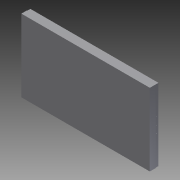
# Autodesk Inventor part: tv
Saved by Autodesk Inventor 2014 (Build 180170000, 170)
## iProperties
Created: 2014-03-21
Part Number: tv
Material: Generic
Document SubType Name: Modeling
Designer: joe_000
Density: 1 g/cm^3
Appearance: Default
largeScrewDiameter: 0.195 in
screwDistanceFromBack: 0.641 in
largeScrewDistance: 5.875 in
topLargeScrewDistanceFromTop: 11.750 in
Author: joe_000
Autodesk Inventor part; units mm, degrees
ref_plane "YZ Plane" through (0, 0, 0) normal (1, 0, 0) x (0, 1, 0)
ref_plane "XZ Plane" through (0, 0, 0) normal (0, 1, 0) x (-1, 0, 0)
ref_plane "XY Plane" through (0, 0, 0) normal (0, 0, 1) x (1, 0, 0)
sketch "Sketch1" plane through (0, 0, 0) normal (0, 0, 1) x (1, 0, 0)
  line L0 (0, 0) -> (1339.85, 0)
  line L1 (1339.85, 0) -> (1339.85, 755.65)
  line L2 (1339.85, 755.65) -> (0, 755.65)
  line L3 (0, 755.65) -> (0, 0)
  dimension "tvWidth" = 1339.85
  dimension "tvHeight" = 755.65
  dimension "tvDiagonal" = 1538.2474
  constraints: 8 end point, 2 parallel, 1 horizontal, 1 perpendicular
  measures "tvWidth" distance of L1.end L2.end
  measures "tvHeight" distance of L0.end L1.end
  measures "tvDiagonal" distance of L1.end L0.start
extrude "Extrusion1" add sketch "Sketch1" against normal blind 59.9281
sketch "Sketch2" plane through (0, 0, -59.9281) normal (0, 0, -1) x (-1, 0, 0)
  line L0 (-1339.85, 0) -> (-1339.85, 755.65) projected
  line L1 (0, 0) -> (-1339.85, 0) projected
  line L2 (0, 755.65) -> (0, 0) projected
  line L3 (-1339.85, 755.65) -> (0, 755.65) projected
  line L4 (-1337.8656, 753.6656) -> (-1.9844, 753.6656)
  line L5 (-1.9844, 753.6656) -> (-1.9844, 1.9844)
  line L6 (-1.9844, 1.9844) -> (-1337.8656, 1.9844)
  line L7 (-1337.8656, 1.9844) -> (-1337.8656, 753.6656)
  dimension "backBezelToFrontBezelSizeDifference" = 1.9844
  dimension "d7" = 1.9844
  dimension "d8" = 1.9844
  dimension "d9" = 1.9844
  constraints: 8 end point, 2 parallel, 1 horizontal, 1 perpendicular
  measures "backBezelToFrontBezelSizeDifference" distance between parallel lines of L2 L5
  measures "d7" distance between parallel lines of L3 L4
  measures "d8" distance between parallel lines of L0 L7
  measures "d9" distance between parallel lines of L1 L6
extrude "Extrusion2" add sketch "Sketch2" along normal blind 32.1469 contours L4 L5 L6 L7
sketch "Sketch3" plane through (1337.8656, 1.9844, -59.9281) normal (1, 0, 0) x (0, 0, -1)
  line L0 (32.1469, 0) -> (32.1469, 751.6812) projected
  line L1 (0, 751.6812) -> (32.1469, 751.6812) projected
  circle A0 centre (15.875, 453.2312) radius 2.4805
  circle A1 centre (15.875, 304.0062) radius 2.4805
  circle A2 centre (15.875, 378.4203) radius 1.6867
  point P0 (-59.9281, -1.9844)
  dimension "largeScrewDistance" = 149.225
  dimension "largeScrewToSmallScrewDistance" = 74.8109
  dimension "screwDistanceFromBack" = 16.2719
  dimension "topLargeScrewDistanceFromTop" = 298.45
  dimension "largeScrewDiameter" = 4.9609
  dimension "smallScrewDiameter" = 3.3734
  constraints: 3 centre point, 2 vertical alignment, 1 equal radius
  measures "largeScrewDistance" distance of A0.centre A1.centre
  measures "largeScrewToSmallScrewDistance" distance of A2.centre A0.centre
  measures "screwDistanceFromBack" distance from line of L0 A0.centre
  measures "topLargeScrewDistanceFromTop" distance from line of L1 A0.centre
  measures "largeScrewDiameter" diameter of A0
  measures "smallScrewDiameter" diameter of A2
extrude "Extrusion3" cut sketch "Sketch3" against normal blind 18.2563
equation "\"d7\" = backBezelToFrontBezelSizeDifference"
equation "\"d8\" = backBezelToFrontBezelSizeDifference"
equation "\"d9\" = backBezelToFrontBezelSizeDifference"
body "Solid1"
